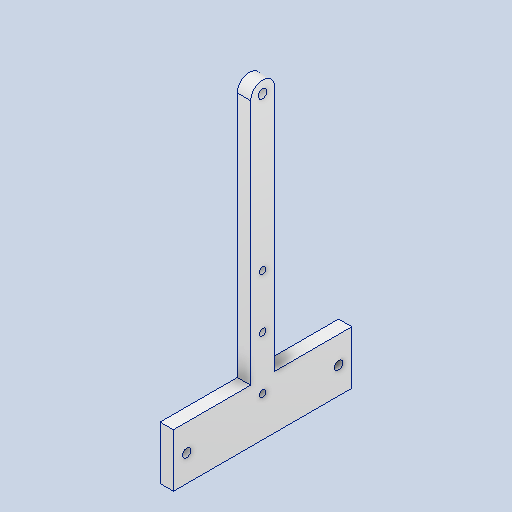
# Autodesk Inventor part: odom_v1_Plate_5
Saved by Autodesk Inventor 2025.2 (Build 292293000, 293)
## iProperties
Created: 2025-04-01
Part Number: odom_v1_Plate_5
Material: アルミニウム 6061
Document SubType Name: Modeling
Designer: haruy
Density: 2.7 g/cm^3
Appearance: アルミニウム - フラット
Author: haruy
Autodesk Inventor part; units mm, degrees
ref_plane "YZ Plane" through (0, 0, 0) normal (1, 0, 0) x (0, 1, 0)
ref_plane "XZ Plane" through (0, 0, 0) normal (0, 1, 0) x (-1, 0, 0)
ref_plane "XY Plane" through (0, 0, 0) normal (0, 0, 1) x (1, 0, 0)
derived "odom_v1_Sketch_Base.ipt"
sketch "スケッチ1" plane through (300, 0, 0) normal (1, 0, 0) x (0, 1, 0)
  line L0 (0, 0) -> (20, 0)
  line L1 (20, 0) -> (20, -192.6893)
  line L2 (20, -192.6893) -> (0, -192.6893)
  line L3 (0, -192.6893) -> (0, 0)
  line L4 (-77, 0) -> (-77, -265.1297)
  circle A0 centre (7.5, -57.9764) radius 1.6
  circle A1 centre (7.5, -93.4764) radius 1.6
  line L5 (-20, -52.2264) -> (-66, -52.2264)
  line L6 (-66, -52.2264) -> (-66, -57.2264)
  line L7 (-66, -57.2264) -> (-20, -57.2264)
  line L8 (-20, -57.2264) -> (-20, -52.2264)
  line L9 (-20, -94.2264) -> (-66, -94.2264)
  line L10 (-66, -94.2264) -> (-66, -99.2264)
  line L11 (-66, -99.2264) -> (-20, -99.2264)
  line L12 (-20, -99.2264) -> (-20, -94.2264)
  line L13 (-19.371, -66.7264) -> (-77, -66.7264)
  line L14 (-77, -66.7264) -> (-77, -84.7264)
  line L15 (-77, -84.7264) -> (-19.371, -84.7264)
  line L16 (-19.371, -84.7264) -> (-19.371, -66.7264)
  line L17 (-41.1855, -57.2264) -> (-55.1855, -57.2264)
  line L18 (-55.1855, -57.2264) -> (-55.1855, -58.0264)
  line L19 (-55.1855, -58.0264) -> (-41.1855, -58.0264)
  line L20 (-41.1855, -58.0264) -> (-41.1855, -57.2264)
  line L21 (-48.1855, -66.7264) -> (-48.1855, -84.7264)
  line L22 (-55.1855, -94.2264) -> (-41.1855, -94.2264)
  line L23 (-41.1855, -94.2264) -> (-41.1855, -93.4264)
  line L24 (-41.1855, -93.4264) -> (-55.1855, -93.4264)
  line L25 (-55.1855, -93.4264) -> (-55.1855, -94.2264)
  circle A2 centre (48, -75.7264) radius 1.65
  circle A3 centre (-17, -75.7264) radius 2
  line L26 (48, -75.7264) -> (-17, -75.7264)
  line L27 (33.5, -67.2264) -> (-12, -67.2264)
  line L28 (-12, -67.2264) -> (-12, -84.2264)
  line L29 (-12, -84.2264) -> (33.5, -84.2264)
  line L30 (33.5, -84.2264) -> (33.5, -67.2264)
  line L31 (-12, -73.7264) -> (-20, -73.7264)
  line L32 (-20, -73.7264) -> (-20, -77.7264)
  line L33 (-20, -77.7264) -> (-12, -77.7264)
  line L34 (-12, -77.7264) -> (-12, -73.7264)
  line L35 (-2, -71.2264) -> (-57, -71.2264)
  line L36 (-57, -71.2264) -> (-57, -80.2264)
  line L37 (-57, -80.2264) -> (-2, -80.2264)
  line L38 (-2, -80.2264) -> (-2, -71.2264)
  circle A4 centre (-9.5, -75.7264) radius 1.25
  circle A5 centre (-29.5, -75.7264) radius 1.25
  circle A6 centre (-49.5, -75.7264) radius 1.25
  line L39 (-52, -65.7264) -> (-22, -65.7264)
  line L40 (-22, -65.7264) -> (-22, -85.7264)
  line L41 (-22, -85.7264) -> (-52, -85.7264)
  line L42 (-52, -85.7264) -> (-52, -65.7264)
  line L43 (-43, -52.2264) -> (-43, -57.2264)
  circle A7 centre (-33, -54.7264) radius 1.25
  line L44 (-29.5, -75.7264) -> (-49.5, -75.7264)
  circle A8 centre (-53, -54.7264) radius 1.25
  circle A9 centre (-53, -96.7264) radius 1.25
  circle A10 centre (-33, -96.7264) radius 1.25
  line L45 (-44.5, -42.2264) -> (-64.5, -42.2264)
  line L46 (-64.5, -42.2264) -> (-64.5, -109.2264)
  line L47 (-64.5, -109.2264) -> (-44.5, -109.2264)
  line L48 (-44.5, -109.2264) -> (-44.5, -42.2264)
  circle A11 centre (-54.5, -47.2264) radius 1.6
  circle A12 centre (-54.5, -104.2264) radius 1.6
  circle A13 centre (48, -75.7264) radius 4.5
  line L49 (48, -71.2264) -> (-2, -71.2264)
  line L50 (-2, -80.2264) -> (48, -80.2264)
  point P0 (-44.5, -71.2264)
  point P1 (-44.5, -80.2264)
  dimension "d1" = 20
  dimension "d2" = 12.5
  dimension "d3" = 3.2
  dimension "d4" = 3.2
  dimension "d5" = 10
  dimension "d7" = 10
  dimension "d10" = 5
  dimension "d11" = 5
  dimension "d12" = 5
  dimension "d13" = 5
  dimension "d14" = 9
  measures "d1" distance of L47.end L46.end
  measures "d2" distance between parallel lines of L4 L46
  measures "d3" diameter of A11
  measures "d4" diameter of A12
  measures "d5" distance from line of A11.centre L46
  measures "d7" distance from line of A12.centre L46
  measures "d10" distance from line of A11.centre L45
  measures "d11" distance from line of L47 A12.centre
  measures "d12" distance from line of L5 A11.centre
  measures "d13" distance from line of A12.centre L11
  measures "d14" diameter of A13
extrude "押し出し1" add sketch "スケッチ1" against normal blind 5 contours L49 L1 L26 L3 | L3 L26 L38 L49 | L49 L30 L26 L1 | L26 L1 L50 L3 | L3 L50 L38 L26 | L38 L26 A4 L28 L35 | L28 L31 L16 L35 | L26 L30 L50 L1 | L49 A13 L26 L30 | L38 L37 L28 L26 A4 | L28 L26 A3 L31 | L16 L31 L32 L33 L37 L40 L35 | L26 A13 L50 L30 | A13 | L28 L33 A3 L26 | A3 | A3 L33 L16 L31 | L16 L33 L32 L31 | L40 L37 L48 L35 | L37 L16 L33 L28 | L48 L44 L21 L35 | L35 L21 L13 L48 | L13 L42 L39 L48 | L35 L42 L13 L21 | L21 L37 L42 L35 | L48 L37 L21 L44 | L48 L15 L21 L37 | L39 L42 L13 L46 L7 L18 L19 L48 | L42 L37 L36 L35 | L35 L36 L37 L42 L15 L46 L13 | L21 L15 L42 L37 | L48 L41 L42 L15 | L19 L18 L7 L48 | L48 L24 L25 L9 L46 L15 L42 L41 | L7 L46 L5 L48 | L48 L9 L25 L24 | L5 L46 L45 L48 | L48 L11 L46 L9 | L48 L47 L46 L11 | A8 | A9
equation "\"d4\" = d3"
